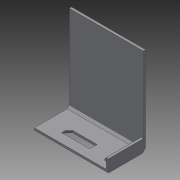
# Autodesk Inventor part: laptop_port_cover
Saved by Autodesk Inventor 2015 (Build 190159000, 159)
## iProperties
Created: 2014-10-07
Part Number: laptop_port_cover
Material: Generic
Document SubType Name: Modeling
Designer: Drew
Density: 1 g/cm^3
Appearance: Default
Author: Drew
Autodesk Inventor part; units mm, degrees
ref_plane "YZ Plane" through (0, 0, 0) normal (1, 0, 0) x (0, 1, 0)
ref_plane "XZ Plane" through (0, 0, 0) normal (0, 1, 0) x (-1, 0, 0)
ref_plane "XY Plane" through (0, 0, 0) normal (0, 0, 1) x (1, 0, 0)
sketch "Sketch1" plane through (0, 0, 0) normal (0, 1, 0) x (-1, 0, 0)
  line L0 (19.75, 23.5) -> (-19.75, 23.5)
  line L1 (-19.75, 23.5) -> (-19.75, -23.5)
  line L2 (-19.75, -23.5) -> (19.75, -23.5)
  line L3 (19.75, -23.5) -> (19.75, 23.5)
  line L4 (0, -28.9451) -> (0, 30.9067)
  line L5 (30.9717, 0) -> (-30.2589, 0)
  point P0 (0, 0)
  dimension "d0" = 39.5
  dimension "d1" = 47
  constraints: 12 end point, 2 horizontal, 2 parallel, 2 point on line, 1 perpendicular, 1 vertical, 2 other
  measures "d0" distance of L1.end L2.end
  measures "d1" distance of L2.end L0.start
extrude "Extrusion1" add sketch "Sketch1" along normal blind 1.15
sketch "Sketch2" plane through (0, 0, 0) normal (0, 1, 0) x (-1, 0, 0)
  line L0 (-18.6, -22.35) -> (-18.6, -16.9)
  line L1 (-18.6, -16.9) -> (-19.75, -16.9)
  line L2 (-19.75, -16.9) -> (-19.75, -23.5)
  line L3 (-19.75, -23.5) -> (19.75, -23.5)
  line L4 (19.75, -23.5) -> (19.75, -22.35)
  line L5 (19.75, -22.35) -> (-18.6, -22.35)
  line L6 (19.75, -23.5) -> (19.75, 23.5) projected
  point P0 (0, 0)
  point P1 (19.75, -22.925)
  dimension "d7" = 6.6
  dimension "d9" = 1.15
  constraints: 12 end point, 2 parallel, 2 perpendicular, 1 horizontal, 1 midpoint, 1 point on line
  measures "d7" distance of L1.end L2.end
  measures "d9" distance of L3.end L4.end
extrude "Extrusion2" add sketch "Sketch2" against normal blind 18.65
chamfer "Chamfer1" distance 1.15 angle 45 1 edges at (-0.575, 0, -22.35) measured on face at (-0.575, -0.5, -22.35)
chamfer "Chamfer3" distance 1.75 angle 45 1 edges at (0, 1.15, -23.5)
sketch "Sketch3" plane through (19.75, -18.65, -23.5) normal (0, 0, -1) x (-1, 0, 0)
  line L0 (30, 5) -> (15, 5)
  line L1 (15, 5) -> (15, 9)
  line L2 (15, 9) -> (28, 9)
  line L3 (30, 7) -> (30, 5)
  circle A0 centre (5, 5) radius 1.5
  line L4 (28, 9) -> (30, 7)
  line L5 (0, 0) -> (0, 18.05) projected
  line L6 (39.5, 0) -> (0, 0) projected
  point P0 (19.75, 18.65)
  dimension "d19" = 3
  dimension "d21" = 135
  dimension "d22" = 135
  dimension "d23" = 15
  dimension "d24" = 15
  dimension "d25" = 4
  dimension "d34" = 5
  dimension "d35" = 5
  dimension "d36" = 5
  dimension "d37" = 13
  constraints: 10 end point, 2 parallel, 1 centre point, 1 horizontal, 1 perpendicular
  measures "d19" diameter of A0
  measures "d21" angle of L2 L4
  measures "d22" angle of L3 L4
  measures "d23" distance between parallel lines of L5 L1
  measures "d24" distance between parallel lines of L1 L3
  measures "d25" distance of L0.end L1.end
  measures "d34" distance from line of A0.centre L5
  measures "d35" distance from line of A0.centre L6
  measures "d36" distance between parallel lines of L0 L6
  measures "d37" distance of L1.end L2.end
extrude "Extrusion3" cut sketch "Sketch3" against normal blind 1.15
body "Solid1"
